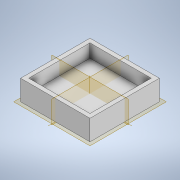
# Autodesk Inventor part: Base
Saved by Autodesk Inventor 2021 (Build 250183000, 183)
## iProperties
Created: 2022-11-29
Part Number: Base
Material: Generisch
Document SubType Name: Modeling
Designer: Elian
Density: 1 g/cm^3
Appearance: Vorgabe
Author: Elian
Autodesk Inventor part; units mm, degrees
sketch "Skizze1" plane through (0, 0, 0) normal (0, 1, 0) x (-1, 0, 0)
  line L0 (34, -34) -> (-34, -34)
  line L1 (-34, -34) -> (-34, 34)
  line L2 (-34, 34) -> (34, 34)
  line L3 (34, 34) -> (34, -34)
  line L4 (0, -47.6) -> (0, 47.6) projected
  line L5 (47.6, 0) -> (-47.6, 0) projected
  point P0 (0, 0)
  dimension "d0" = 68
  dimension "d1" = 68
  constraints: 8 end point, 2 parallel, 1 horizontal, 1 perpendicular, 2 other
  measures "d0" distance of L0.end L1.end
  measures "d1" distance of L0.start L0.end
extrude "Extrusion1" add sketch "Skizze1" along normal blind 20
sketch "Skizze2" plane through (0, 20, 0) normal (0, 1, 0) x (1, 0, 0)
  line L0 (-30, 30) -> (30, 30)
  line L1 (30, 30) -> (30, -30)
  line L2 (30, -30) -> (-30, -30)
  line L3 (-30, -30) -> (-30, 30)
  line L4 (-47.6, 0) -> (47.6, 0) projected
  line L5 (0, 47.6) -> (0, -47.6) projected
  line L6 (-34, 34) -> (-34, -34) projected
  line L7 (34, -34) -> (34, 34) projected
  point P0 (0, 0)
  dimension "d4" = 60
  dimension "d5" = 60
  dimension "d6" = 4
  dimension "d7" = 4
  constraints: 8 end point, 2 parallel, 1 horizontal, 1 perpendicular, 2 other
  measures "d4" distance of L1.end L2.end
  measures "d5" distance of L0.end L1.end
  measures "d6" distance between parallel lines of L6 L3
  measures "d7" distance between parallel lines of L7 L1
extrude "Extrusion2" cut sketch "Skizze2" against normal blind 13
sketch "Skizze4" plane through (0, 0, 0) normal (0, -1, 0) x (1, 0, 0)
  line L0 (0, 12) -> (0, -12) construction
  line L1 (-2, 12) -> (-2, -12)
  line L2 (2, -12) -> (2, 12)
  arc A0 (2, 12) -> (-2, 12) centre (0, 12) ccw
  arc A1 (-2, -12) -> (2, -12) centre (0, -12) ccw
  line L3 (-47.6, 0) -> (47.6, 0) projected
  line L4 (12, 0) -> (-12, 0) construction
  line L5 (12, 2) -> (-12, 2)
  line L6 (-12, -2) -> (12, -2)
  arc A2 (12, -2) -> (12, 2) centre (12, 0) ccw
  arc A3 (-12, 2) -> (-12, -2) centre (-12, 0) ccw
  line L7 (0, -47.6) -> (0, 47.6) projected
  line L8 (-3.0851, 4.7663) -> (-2, 12)
  line L9 (3.0851, 4.7663) -> (2, 12)
  line L10 (-3.0851, -4.7663) -> (-2, -12)
  line L11 (3.0851, -4.7663) -> (2, -12)
  line L12 (-4.7663, 3.0851) -> (-12, 2)
  line L13 (-4.7663, -3.0851) -> (-12, -2)
  line L14 (4.7663, 3.0851) -> (12, 2)
  line L15 (4.7663, -3.0851) -> (12, -2)
  arc A4 (-4.7663, 3.0851) -> (-3.0851, 4.7663) centre (-5.0629, 5.0629) ccw
  arc A5 (3.0851, 4.7663) -> (4.7663, 3.0851) centre (5.0629, 5.0629) ccw
  arc A6 (4.7663, -3.0851) -> (3.0851, -4.7663) centre (5.0629, -5.0629) ccw
  arc A7 (-3.0851, -4.7663) -> (-4.7663, -3.0851) centre (-5.0629, -5.0629) ccw
  point P0 (0, 0)
  point P1 (0, 0)
  point P2 (0, 0)
  point P3 (-3.5, 2)
  point P4 (3.5, 2)
  point P5 (-3.5, -2)
  point P6 (3.5, -2)
  point P7 (-2, 3.5)
  point P8 (-2, -3.5)
  point P9 (2, 3.5)
  point P10 (2, -3.5)
  dimension "d30" = 4
  dimension "d31" = 24
  dimension "d32" = 2
  dimension "d33" = 4
  dimension "d34" = 24
  dimension "d35" = 2
  dimension "d36" = 2
  constraints: 32 end point, 18 point on circle, 16 tangent, 12 point on line, 12 symmetric about line, 8 centre point, 2 equal radius, 2 midpoint, 2 parallel, 1 vertical, 2 other
  measures "d30" diameter of A1
  measures "d31" distance of L0.end L0.start
  measures "d32" radius of A0
  measures "d33" diameter of A3
  measures "d34" distance of L6.start L6.end
  measures "d35" radius of A4
  measures "d36" radius of A6
extrude "Extrusion4" cut sketch "Skizze4" against normal blind 3
